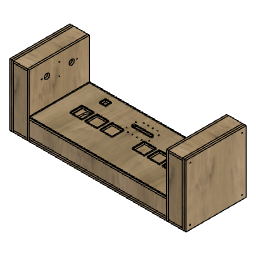
ongekicon-diy (Autodesk Fusion 360 design; units mm, degrees)
Autodesk Fusion 360 part; units mm, degrees
(part 1 of 3)
sketch "스케치1" plane through (0, 0, 0) normal (0, 0, 1) x (1, 0, 0)
  line L0 (289, -642.7336) -> (375, -642.7336)
  line L1 (375, -656.7336) -> (289, -656.7336)
  arc A0 (289, -642.7336) -> (289, -656.7336) centre (289, -649.7336) ccw
  arc A1 (375, -656.7336) -> (375, -642.7336) centre (375, -649.7336) ccw
  line L2 (289, -642.7336) -> (289, -656.7336) construction
  line L3 (375, -642.7336) -> (375, -656.7336) construction
  line L4 (375, -642.7336) -> (386.9217, -626.4866) construction
  line L5 (386.9217, -626.4866) -> (386.9217, -642.6701) construction
  line L6 (386.9217, -642.6701) -> (386.9217, -656.6701) construction
  line L7 (386.9217, -656.6701) -> (386.9217, -672.8535) construction
  line L8 (375, -656.7336) -> (386.9217, -672.8535) construction
  line L9 (386.9217, -642.6701) -> (386.9217, -656.6701) construction
  line L10 (375, -642.7336) -> (375, -656.7336) construction
  line L11 (375, -642.7336) -> (386.9217, -626.4866) construction
  line L12 (375, -656.7336) -> (386.9217, -672.8535) construction
  line L13 (386.9217, -656.6701) -> (386.9217, -672.8535) construction
  line L14 (386.9217, -626.4866) -> (386.9217, -642.6701) construction
  arc A2 (375, -656.7336) -> (375, -642.7336) centre (375, -649.7336) ccw
  line L15 (375, -642.7336) -> (386.9217, -642.7336) construction
  line L16 (289, -642.7336) -> (277.0783, -642.7336) construction
  line L17 (277.0783, -642.7336) -> (277.0783, -626.5501) construction
  line L18 (277.0783, -626.5501) -> (289, -642.7336) construction
  line L19 (289, -656.7336) -> (277.0783, -656.7336) construction
  line L20 (277.0783, -656.7336) -> (277.0783, -672.9171) construction
  line L21 (289, -656.7336) -> (277.0783, -672.9171) construction
  circle A3 centre (277.0783, -626.5501) radius 2.65
  circle A4 centre (277.0783, -672.9171) radius 2.65
  circle A5 centre (386.9217, -626.4866) radius 2.65
  circle A6 centre (386.9217, -672.8535) radius 2.65
  line L22 (299.0783, -611.6097) -> (277.0783, -626.5501) construction
  circle A7 centre (299.0783, -611.6097) radius 2.65
  line L23 (299.0783, -611.6097) -> (321.0783, -611.6097) construction
  line L24 (321.0783, -611.6097) -> (343.0783, -611.6097) construction
  line L25 (343.0783, -611.6097) -> (365.0783, -611.6097) construction
  line L26 (364.9217, -687.7939) -> (386.9217, -672.8535) construction
  line L27 (364.9217, -687.7939) -> (342.9217, -687.7939) construction
  line L28 (342.9217, -687.7939) -> (320.9217, -687.7939) construction
  line L29 (320.9217, -687.7939) -> (298.9217, -687.7939) construction
  circle A8 centre (321.0783, -611.6097) radius 2.65
  circle A9 centre (343.0783, -611.6097) radius 2.65
  circle A10 centre (365.0783, -611.6097) radius 2.65
  circle A11 centre (364.9217, -687.7939) radius 2.65
  circle A12 centre (342.9217, -687.7939) radius 2.65
  circle A13 centre (320.9217, -687.7939) radius 2.65
  circle A14 centre (298.9217, -687.7939) radius 2.65
  line L30 (0, -575) -> (664, -575)
  line L31 (664, -575) -> (664, -866)
  line L32 (664, -866) -> (0, -866)
  line L33 (0, -866) -> (0, -575)
  line L34 (0, -575) -> (332, -575) construction
  line L35 (332, -575) -> (332, -649.7336) construction
  line L36 (0, -649.7336) -> (0, -575) construction
  line L37 (332, -649.7336) -> (289, -649.7336) construction
  line L38 (150.8081, -749.0793) -> (137.915, -749.0793) construction
  line L39 (223.7013, -749.0793) -> (210.8081, -749.0793) construction
  line L40 (842.8371, -502.2992) -> (842.8371, -516.2992) construction
  line L41 (820.8371, -547.4231) -> (842.8371, -532.4827) construction
  line L42 (830.9154, -502.3627) -> (830.9154, -516.3627) construction
  line L43 (830.9154, -516.3627) -> (842.8371, -532.4827) construction
  line L44 (842.8371, -516.2992) -> (842.8371, -532.4827) construction
  circle A15 centre (798.8371, -547.4231) radius 2.65
  circle A16 centre (798.9937, -471.2388) radius 2.65
  line L45 (798.9937, -471.2388) -> (820.9937, -471.2388) construction
  circle A17 centre (820.8371, -547.4231) radius 2.65
  circle A18 centre (842.8371, -532.4827) radius 2.65
  line L46 (820.8371, -547.4231) -> (798.8371, -547.4231) construction
  circle A19 centre (842.8371, -486.1157) radius 2.65
  arc A20 (830.9154, -516.3627) -> (830.9154, -502.3627) centre (830.9154, -509.3627) ccw
  circle A21 centre (820.9937, -471.2388) radius 2.65
  line L47 (830.9154, -502.3627) -> (842.8371, -502.3627) construction
  line L48 (830.9154, -502.3627) -> (830.9154, -516.3627) construction
  line L49 (830.9154, -516.3627) -> (842.8371, -532.4827) construction
  arc A22 (830.9154, -516.3627) -> (830.9154, -502.3627) centre (830.9154, -509.3627) ccw
  line L50 (798.8371, -547.4231) -> (776.8371, -547.4231) construction
  line L51 (744.9154, -502.3627) -> (830.9154, -502.3627)
  line L52 (776.9937, -471.2388) -> (798.9937, -471.2388) construction
  line L53 (830.9154, -516.3627) -> (744.9154, -516.3627)
  circle A23 centre (754.8371, -547.4231) radius 2.65
  line L54 (732.9937, -502.3627) -> (732.9937, -486.1792) construction
  circle A24 centre (776.8371, -547.4231) radius 2.65
  line L55 (787.9154, -509.3627) -> (744.9154, -509.3627) construction
  line L56 (744.9154, -502.3627) -> (732.9937, -502.3627) construction
  line L57 (754.9937, -471.2388) -> (776.9937, -471.2388) construction
  circle A25 centre (776.9937, -471.2388) radius 2.65
  circle A26 centre (754.9937, -471.2388) radius 2.65
  line L58 (732.9937, -486.1792) -> (744.9154, -502.3627) construction
  circle A27 centre (732.9937, -532.5462) radius 2.65
  line L59 (776.8371, -547.4231) -> (754.8371, -547.4231) construction
  line L60 (744.9154, -516.3627) -> (732.9937, -516.3627) construction
  line L61 (732.9937, -516.3627) -> (732.9937, -532.5462) construction
  line L62 (754.9937, -471.2388) -> (732.9937, -486.1792) construction
  line L63 (744.9154, -502.3627) -> (744.9154, -516.3627) construction
  line L64 (830.9154, -502.3627) -> (842.8371, -486.1157) construction
  line L65 (842.8371, -486.1157) -> (842.8371, -502.2992) construction
  line L66 (842.8371, -516.2992) -> (842.8371, -532.4827) construction
  line L67 (842.8371, -486.1157) -> (842.8371, -502.2992) construction
  line L68 (842.8371, -502.2992) -> (842.8371, -516.2992) construction
  line L69 (830.9154, -502.3627) -> (842.8371, -486.1157) construction
  line L70 (744.9154, -516.3627) -> (732.9937, -532.5462) construction
  circle A28 centre (732.9937, -486.1792) radius 2.65
  arc A29 (744.9154, -502.3627) -> (744.9154, -516.3627) centre (744.9154, -509.3627) ccw
  circle A30 centre (-55.9858, -345.9527) radius 2.65
  line L71 (-55.9858, -299.5858) -> (-55.9858, -315.7693) construction
  circle A31 centre (-77.8292, -284.7089) radius 2.65
  line L72 (-153.9075, -329.8328) -> (-165.8292, -346.0163) construction
  line L73 (-121.8292, -284.7089) -> (-99.8292, -284.7089) construction
  line L74 (-153.9075, -329.8328) -> (-165.8292, -329.8328) construction
  arc A32 (-153.9075, -315.8328) -> (-153.9075, -329.8328) centre (-153.9075, -322.8328) ccw
  line L75 (-165.8292, -329.8328) -> (-165.8292, -346.0163) construction
  circle A33 centre (-165.8292, -299.6493) radius 2.65
  circle A34 centre (-143.9858, -360.8931) radius 2.65
  line L76 (-143.8292, -284.7089) -> (-121.8292, -284.7089) construction
  line L77 (-153.9075, -315.8328) -> (-153.9075, -329.8328) construction
  line L78 (-153.9075, -315.8328) -> (-165.8292, -315.8328) construction
  circle A35 centre (-121.8292, -284.7089) radius 2.65
  line L79 (-67.9075, -329.8328) -> (-153.9075, -329.8328)
  line L80 (-55.9858, -315.7693) -> (-55.9858, -329.7693) construction
  line L81 (-153.9075, -315.8328) -> (-67.9075, -315.8328)
  circle A36 centre (-77.9858, -360.8931) radius 2.65
  arc A37 (-67.9075, -329.8328) -> (-67.9075, -315.8328) centre (-67.9075, -322.8328) ccw
  arc A38 (-67.9075, -329.8328) -> (-67.9075, -315.8328) centre (-67.9075, -322.8328) ccw
  line L82 (-67.9075, -315.8328) -> (-55.9858, -299.5858) construction
  line L83 (-67.9075, -315.8328) -> (-67.9075, -329.8328) construction
  line L84 (-67.9075, -315.8328) -> (-55.9858, -315.8328) construction
  circle A39 centre (-55.9858, -299.5858) radius 2.65
  line L85 (-99.8292, -284.7089) -> (-77.8292, -284.7089) construction
  line L86 (-67.9075, -329.8328) -> (-55.9858, -345.9527) construction
  circle A40 centre (-99.9858, -360.8931) radius 2.65
  line L87 (-77.9858, -360.8931) -> (-55.9858, -345.9527) construction
  circle A41 centre (-99.8292, -284.7089) radius 2.65
  line L88 (-55.9858, -299.5858) -> (-55.9858, -315.7693) construction
  line L89 (-67.9075, -329.8328) -> (-55.9858, -345.9527) construction
  line L90 (-77.9858, -360.8931) -> (-99.9858, -360.8931) construction
  line L91 (-55.9858, -329.7693) -> (-55.9858, -345.9527) construction
  line L92 (-55.9858, -329.7693) -> (-55.9858, -345.9527) construction
  line L93 (-165.8292, -315.8328) -> (-165.8292, -299.6493) construction
  line L94 (-165.8292, -299.6493) -> (-153.9075, -315.8328) construction
  line L95 (-99.9858, -360.8931) -> (-121.9858, -360.8931) construction
  line L96 (-110.9075, -322.8328) -> (-153.9075, -322.8328) construction
  circle A42 centre (-165.8292, -346.0163) radius 2.65
  line L97 (-121.9858, -360.8931) -> (-143.9858, -360.8931) construction
  line L98 (-67.9075, -315.8328) -> (-55.9858, -299.5858) construction
  line L99 (-67.9075, -315.8328) -> (-67.9075, -329.8328) construction
  circle A43 centre (-143.8292, -284.7089) radius 2.65
  circle A44 centre (-121.9858, -360.8931) radius 2.65
  line L100 (-55.9858, -315.7693) -> (-55.9858, -329.7693) construction
  line L101 (-143.8292, -284.7089) -> (-165.8292, -299.6493) construction
  line L102 (0, -1260) -> (664, -1260)
  line L103 (664, -1260) -> (664, -1333)
  line L104 (664, -1333) -> (0, -1333)
  line L105 (0, -1333) -> (0, -1260)
  line L106 (0, -1495) -> (0, -1422)
  line L107 (664, -1422) -> (664, -1495)
  line L108 (0, -1422) -> (664, -1422)
  line L109 (664, -1495) -> (0, -1495)
  circle A45 centre (-680.319, -279.9365) radius 2.65
  line L110 (-604.942, -341.2219) -> (-664.942, -341.2219)
  circle A46 centre (-658.319, -264.9961) radius 2.65
  line L111 (-592.0489, -341.2219) -> (-604.942, -341.2219) construction
  line L112 (-834.4326, -341.2219) -> (-834.4326, -281.2219)
  line L113 (-907.3257, -341.2219) -> (-967.3257, -341.2219)
  line L114 (-592.0489, -281.2219) -> (-532.0489, -281.2219)
  line L115 (-967.3257, -281.2219) -> (-907.3257, -281.2219)
  line L116 (-761.5395, -281.2219) -> (-821.5395, -281.2219)
  line L117 (-907.3257, -281.2219) -> (-907.3257, -341.2219)
  line L118 (-821.5395, -341.2219) -> (-834.4326, -341.2219) construction
  line L119 (-532.0489, -341.2219) -> (-592.0489, -341.2219)
  line L120 (-821.5395, -341.2219) -> (-761.5395, -341.2219)
  line L121 (-1045.2407, -198.34) -> (-1045.2407, -167.1425) construction
  line L122 (-821.5395, -281.2219) -> (-821.5395, -341.2219)
  line L123 (-894.4326, -281.2219) -> (-894.4326, -341.2219)
  line L124 (-967.3257, -341.2219) -> (-967.3257, -281.2219)
  circle A47 centre (-724.1625, -203.7522) radius 2.65
  circle A48 centre (-746.1625, -203.7522) radius 2.65
  circle A49 centre (-724.319, -279.9365) radius 2.65
  arc A50 (-756.2407, -234.8761) -> (-756.2407, -248.8761) centre (-756.2407, -241.8761) ccw
  line L125 (-761.5395, -341.2219) -> (-761.5395, -281.2219)
  circle A51 centre (-680.1625, -203.7522) radius 2.65
  line L126 (-592.0489, -341.2219) -> (-592.0489, -281.2219)
  circle A52 centre (-768.1625, -265.0596) radius 2.65
  circle A53 centre (-746.319, -279.9365) radius 2.65
  line L127 (-670.2407, -248.8761) -> (-756.2407, -248.8761)
  circle A54 centre (-768.1625, -218.6926) radius 2.65
  line L128 (-756.2407, -234.8761) -> (-670.2407, -234.8761)
  line L129 (-381.2407, -167.1425) -> (-381.2407, -198.34) construction
  line L130 (-903.551, -198.34) -> (-903.551, -231.34)
  line L131 (-903.551, -231.34) -> (-936.551, -231.34)
  line L132 (-894.4326, -341.2219) -> (-834.4326, -341.2219)
  line L133 (-894.4326, -341.2219) -> (-907.3257, -341.2219) construction
  line L134 (-1045.2407, -241.8761) -> (-1045.2407, -167.1425) construction
  line L135 (-936.551, -198.34) -> (-903.551, -198.34)
  line L136 (-1045.2407, -167.1425) -> (-381.2407, -167.1425)
  line L137 (-1045.2407, -167.1425) -> (-713.2407, -167.1425) construction
  line L138 (-936.551, -231.34) -> (-936.551, -198.34)
  line L139 (-381.2407, -458.1425) -> (-1045.2407, -458.1425)
  line L140 (-1045.2407, -458.1425) -> (-1045.2407, -167.1425)
  line L141 (-834.4326, -281.2219) -> (-894.4326, -281.2219)
  line L142 (-522.9305, -198.34) -> (-522.9305, -231.34)
  line L143 (-519.1557, -281.2219) -> (-519.1557, -341.2219)
  line L144 (-519.1557, -341.2219) -> (-532.0489, -341.2219) construction
  line L145 (-459.1557, -281.2219) -> (-519.1557, -281.2219)
  line L146 (-519.1557, -341.2219) -> (-459.1557, -341.2219)
  line L147 (-489.9305, -231.34) -> (-489.9305, -198.34)
  line L148 (-532.0489, -281.2219) -> (-532.0489, -341.2219)
  line L149 (-489.9305, -198.34) -> (-522.9305, -198.34)
  line L150 (-522.9305, -231.34) -> (-489.9305, -231.34)
  line L151 (-459.1557, -341.2219) -> (-459.1557, -281.2219)
  line L152 (-381.2407, -167.1425) -> (-381.2407, -458.1425)
  circle A55 centre (-658.319, -218.6291) radius 2.65
  line L153 (-664.942, -281.2219) -> (-604.942, -281.2219)
  line L154 (-664.942, -341.2219) -> (-664.942, -281.2219)
  arc A56 (-670.2407, -248.8761) -> (-670.2407, -234.8761) centre (-670.2407, -241.8761) ccw
  circle A57 centre (-702.1625, -203.7522) radius 2.65
  line L155 (-604.942, -281.2219) -> (-604.942, -341.2219)
  circle A58 centre (-702.319, -279.9365) radius 2.65
  arc A59 (-670.2407, -248.8761) -> (-670.2407, -234.8761) centre (-670.2407, -241.8761) ccw
  line L156 (664, 150) -> (664, -141)
  line L157 (0, -141) -> (0, 150)
  line L158 (664, -141) -> (0, -141)
  line L159 (604, 120) -> (60, 120)
  line L160 (634, -81) -> (634, 90)
  line L161 (30, 90) -> (30, -81)
  line L162 (634, 120) -> (30, -111) construction
  line L163 (60, -111) -> (604, -111)
  line L164 (0, 150) -> (664, 150)
  line L165 (30, 120) -> (634, -111) construction
  line L166 (0, 120) -> (0, 150) construction
  line L167 (664, -141) -> (644.0002, -121.0002) construction
  line L168 (664, 150) -> (644.0002, 130.0002) construction
  line L169 (0, 150) -> (19.9998, 130.0002) construction
  line L170 (0, -141) -> (19.9998, -121.0002) construction
  line L171 (664, -491) -> (644.0002, -471.0002) construction
  line L172 (664, -200) -> (644.0002, -219.9998) construction
  line L173 (634, -431) -> (634, -260)
  line L174 (664, -200) -> (664, -491)
  line L175 (30, -230) -> (634, -461) construction
  line L176 (0, -200) -> (664, -200)
  line L177 (60, -461) -> (604, -461)
  line L178 (664, -491) -> (0, -491)
  line L179 (634, -230) -> (30, -461) construction
  line L180 (30, -260) -> (30, -431)
  line L181 (0, -491) -> (19.9998, -471.0002) construction
  line L182 (604, -230) -> (60, -230)
  line L183 (0, -491) -> (0, -200)
  line L184 (0, -200) -> (19.9998, -219.9998) construction
  line L185 (0, -230) -> (0, -200) construction
  arc A60 (60, 120) -> (30, 90) centre (60, 90) ccw
  arc A61 (634, 90) -> (604, 120) centre (604, 90) ccw
  arc A62 (604, -111) -> (634, -81) centre (604, -81) ccw
  arc A63 (30, -81) -> (60, -111) centre (60, -81) ccw
  arc A64 (60, -230) -> (30, -260) centre (60, -260) ccw
  arc A65 (634, -260) -> (604, -230) centre (604, -260) ccw
  arc A66 (604, -461) -> (634, -431) centre (604, -431) ccw
  arc A67 (30, -431) -> (60, -461) centre (60, -431) ccw
  circle A68 centre (644.0002, -219.9998) radius 3.25
  circle A69 centre (644.0002, -471.0002) radius 3.25
  circle A70 centre (644.0002, -121.0002) radius 9
  circle A71 centre (644.0002, 130.0002) radius 9
  circle A72 centre (19.9998, 130.0002) radius 9
  circle A73 centre (19.9998, -121.0002) radius 9
  circle A74 centre (19.9998, -219.9998) radius 3.25
  circle A75 centre (19.9998, -471.0002) radius 3.25
  line L186 (664, -575) -> (644, -575) construction
  line L187 (644, -575) -> (644, -595) construction
  line L188 (644, -595) -> (664, -595) construction
  line L189 (664, -595) -> (664, -575) construction
  line L190 (664, -866) -> (644, -866) construction
  line L191 (644, -866) -> (644, -846) construction
  line L192 (644, -846) -> (664, -846) construction
  line L193 (664, -846) -> (664, -866) construction
  line L194 (0, -866) -> (20, -866) construction
  line L195 (20, -866) -> (20, -846) construction
  line L196 (20, -846) -> (0, -846) construction
  line L197 (0, -846) -> (0, -866) construction
  line L198 (0, -575) -> (20, -575) construction
  line L199 (20, -575) -> (20, -595) construction
  line L200 (20, -595) -> (0, -595) construction
  line L201 (0, -595) -> (0, -575) construction
  circle A76 centre (20, -595) radius 2.5 construction
  circle A77 centre (644, -595) radius 2.5 construction
  circle A78 centre (20, -846) radius 2.5 construction
  circle A79 centre (644, -846) radius 2.5 construction
  line L202 (1066.4968, -1645.2647) -> (1357.4968, -1645.2647)
  line L203 (1357.4968, -1645.2647) -> (1357.4968, -1712.2647)
  line L204 (1357.4968, -1712.2647) -> (1066.4968, -1712.2647)
  line L205 (1066.4968, -1712.2647) -> (1066.4968, -1645.2647)
  line L206 (716.4968, -1645.2647) -> (1007.4968, -1645.2647)
  line L207 (1007.4968, -1645.2647) -> (1007.4968, -1712.2647)
  line L208 (1007.4968, -1712.2647) -> (716.4968, -1712.2647)
  line L209 (716.4968, -1712.2647) -> (716.4968, -1645.2647)
  line L210 (1066.4968, -845.2647) -> (1357.4968, -845.2647)
  line L211 (1357.4968, -845.2647) -> (1357.4968, -912.2647)
  line L212 (1357.4968, -912.2647) -> (1066.4968, -912.2647)
  line L213 (1066.4968, -912.2647) -> (1066.4968, -845.2647)
  line L214 (716.4968, -845.2647) -> (1007.4968, -845.2647)
  line L215 (1007.4968, -845.2647) -> (1007.4968, -912.2647)
  line L216 (1007.4968, -912.2647) -> (716.4968, -912.2647)
  line L217 (716.4968, -912.2647) -> (716.4968, -845.2647)
  line L218 (1406.0943, -1345.433) -> (1473.0943, -1345.433)
  line L219 (1473.0943, -1345.433) -> (1473.0943, -1627.433)
  line L220 (1473.0943, -1627.433) -> (1406.0943, -1627.433)
  line L221 (1406.0943, -1627.433) -> (1406.0943, -1345.433)
  line L222 (1573.0943, -1627.433) -> (1506.0943, -1627.433)
  line L223 (1506.0943, -1627.433) -> (1506.0943, -1345.433)
  line L224 (1506.0943, -1345.433) -> (1573.0943, -1345.433)
  line L225 (1573.0943, -1345.433) -> (1573.0943, -1627.433)
  line L226 (1506.0943, -1277.433) -> (1506.0943, -995.433)
  line L227 (1506.0943, -995.433) -> (1573.0943, -995.433)
  line L228 (1573.0943, -995.433) -> (1573.0943, -1277.433)
  line L229 (1573.0943, -1277.433) -> (1506.0943, -1277.433)
  line L230 (1406.0943, -1277.433) -> (1406.0943, -995.433)
  line L231 (1406.0943, -995.433) -> (1473.0943, -995.433)
  line L232 (1473.0943, -1277.433) -> (1406.0943, -1277.433)
  line L233 (1473.0943, -995.433) -> (1473.0943, -1277.433)
  line L234 (1339.5, -433) -> (1368.5, -433)
  line L235 (1219.5, -433) -> (1248.5, -433)
  line L236 (1248.5, -433) -> (1248.5, -479)
  arc A80 (1370, -497) -> (1385, -482) centre (1370, -482) ccw
  circle A81 centre (1209, -456) radius 2.2592
  line L237 (1203, -415) -> (1385, -497) construction
  arc A82 (1218, -412) -> (1200, -430) centre (1218, -430) ccw
  arc A83 (1218, -415) -> (1203, -430) centre (1218, -430) ccw
  arc A84 (1203, -482) -> (1218, -497) centre (1218, -482) ccw
  line L238 (1218, -497) -> (1370, -497)
  line L239 (1218, -500) -> (1370, -500)
  line L240 (1388, -412) -> (1200, -500) construction
  line L241 (1248.5, -479) -> (1219.5, -479)
  arc A85 (1388, -430) -> (1370, -412) centre (1370, -430) ccw
  circle A86 centre (1294, -486) radius 2.2361
  line L242 (1200, -412) -> (1388, -500) construction
  line L243 (1203, -430) -> (1203, -482)
  line L244 (1370, -415) -> (1218, -415)
  circle A87 centre (1294, -426) radius 2.2361
  line L245 (1370, -412) -> (1218, -412)
  line L246 (1385, -415) -> (1203, -497) construction
  line L247 (1388, -482) -> (1388, -430)
  line L248 (1219.5, -479) -> (1219.5, -433)
  arc A88 (1370, -500) -> (1388, -482) centre (1370, -482) ccw
  arc A89 (1200, -482) -> (1218, -500) centre (1218, -482) ccw
  line L249 (1339.5, -479) -> (1339.5, -433)
  line L250 (1200, -430) -> (1200, -482)
  arc A90 (1385, -430) -> (1370, -415) centre (1370, -430) ccw
  line L251 (1385, -482) -> (1385, -430)
  line L252 (1368.5, -433) -> (1368.5, -479)
  circle A91 centre (1379, -456) radius 2.2361
  line L253 (1368.5, -479) -> (1339.5, -479)
  circle A92 centre (1661.9968, -422.7804) radius 2.2361
  arc A93 (1585.9968, -408.7804) -> (1567.9968, -426.7804) centre (1585.9968, -426.7804) ccw
  line L254 (1587.4968, -429.7804) -> (1616.4968, -429.7804)
  circle A94 centre (1601.9968, -452.7804) radius 12.5
  circle A95 centre (1661.9968, -482.7804) radius 2.2361
  line L255 (1587.4968, -429.7804) -> (1616.4968, -475.7804) construction
  line L256 (1570.9968, -426.7804) -> (1570.9968, -478.7804)
  line L257 (1587.4968, -475.7804) -> (1587.4968, -429.7804)
  line L258 (1616.4968, -475.7804) -> (1587.4968, -475.7804)
  line L259 (1616.4968, -429.7804) -> (1616.4968, -475.7804)
  line L260 (1567.9968, -426.7804) -> (1567.9968, -478.7804)
  line L261 (1516.4968, -587.7804) -> (1516.4968, -660.7804)
  circle A96 centre (1721.9968, -452.7804) radius 12.5
  line L262 (1707.4968, -429.7804) -> (1736.4968, -475.7804) construction
  arc A97 (1752.9968, -426.7804) -> (1737.9968, -411.7804) centre (1737.9968, -426.7804) ccw
  circle A98 centre (1746.9968, -452.7804) radius 2.2361
  line L263 (1707.4968, -475.7804) -> (1707.4968, -429.7804)
  arc A99 (1755.9968, -426.7804) -> (1737.9968, -408.7804) centre (1737.9968, -426.7804) ccw
  arc A100 (1737.9968, -493.7804) -> (1752.9968, -478.7804) centre (1737.9968, -478.7804) ccw
  line L264 (1807.4968, -587.7804) -> (1807.4968, -507.7804) construction
  line L265 (1736.4968, -429.7804) -> (1707.4968, -475.7804) construction
  line L266 (1736.4968, -475.7804) -> (1707.4968, -475.7804)
  arc A101 (1737.9968, -496.7804) -> (1755.9968, -478.7804) centre (1737.9968, -478.7804) ccw
  line L267 (1752.9968, -478.7804) -> (1752.9968, -426.7804)
  line L268 (1707.4968, -429.7804) -> (1736.4968, -429.7804)
  line L269 (1736.4968, -429.7804) -> (1736.4968, -475.7804)
  line L270 (1755.9968, -478.7804) -> (1755.9968, -426.7804)
  circle A102 centre (1576.9968, -452.7804) radius 2.2592
  line L271 (1807.4968, -660.7804) -> (1807.4968, -587.7804)
  arc A103 (1585.9968, -411.7804) -> (1570.9968, -426.7804) centre (1585.9968, -426.7804) ccw
  line L272 (1525.4968, -644.7804) -> (1525.4968, -660.7804) construction
  circle A104 centre (1616.4968, -615.7804) radius 4
  line L273 (1525.4968, -660.7804) -> (1516.4968, -660.7804)
  arc A105 (1570.9968, -626.2804) -> (1574.9968, -630.2804) centre (1570.9968, -630.2804) ccw
  circle A106 centre (1616.4968, -644.7804) radius 4
  line L274 (1585.9968, -496.7804) -> (1737.9968, -496.7804)
  line L275 (1585.9968, -493.7804) -> (1737.9968, -493.7804)
  line L276 (1737.9968, -411.7804) -> (1585.9968, -411.7804)
  line L277 (1807.4968, -378.7804) -> (1516.4968, -378.7804)
  arc A107 (1567.9968, -478.7804) -> (1585.9968, -496.7804) centre (1585.9968, -478.7804) ccw
  arc A108 (1570.9968, -478.7804) -> (1585.9968, -493.7804) centre (1585.9968, -478.7804) ccw
  line L278 (1616.4968, -429.7804) -> (1587.4968, -475.7804) construction
  line L279 (1807.4968, -507.7804) -> (1516.4968, -397.7804) construction
  line L280 (1807.4968, -587.7804) -> (1516.4968, -587.7804)
  line L281 (1737.9968, -408.7804) -> (1585.9968, -408.7804)
  line L282 (1807.4968, -397.7804) -> (1516.4968, -507.7804) construction
  circle A109 centre (1707.4968, -615.7804) radius 4
  line L283 (1516.4968, -660.7804) -> (1807.4968, -660.7804)
  arc A110 (1574.9968, -630.2804) -> (1570.9968, -626.2804) centre (1570.9968, -630.2804) ccw
  circle A111 centre (1707.4968, -644.7804) radius 4
  line L284 (1807.4968, -378.7804) -> (1807.4968, -660.7804)
  line L285 (1516.4968, -378.7804) -> (1516.4968, -660.7804)
  line L286 (1798.4968, -660.7804) -> (1807.4968, -660.7804)
  line L287 (1798.4968, -660.7804) -> (1525.4968, -660.7804)
  circle A112 centre (1661.9968, -630.2804) radius 4
  circle A113 centre (1752.9968, -630.2804) radius 4
  line L288 (725.4968, -1278.433) -> (716.4968, -1278.433)
  line L289 (998.4968, -1278.433) -> (725.4968, -1278.433)
  line L290 (998.4968, -1278.433) -> (1007.4968, -1278.433)
  line L291 (1007.4968, -978.433) -> (1007.4968, -1278.433)
  line L292 (1007.4968, -978.433) -> (716.4968, -978.433)
  line L293 (716.4968, -978.433) -> (716.4968, -1278.433)
  arc A114 (1661.5009, -1535.9592) -> (1691.5009, -1565.9592) centre (1691.5009, -1535.9592) ccw
  line L294 (1871.5009, -1325.9592) -> (1691.5009, -1325.9592)
  arc A115 (1691.5009, -1325.9592) -> (1661.5009, -1355.9592) centre (1691.5009, -1355.9592) ccw
  line L295 (1661.5009, -1355.9592) -> (1661.5009, -1535.9592)
  circle A116 centre (1656.0009, -1571.4592) radius 3.25
  circle A117 centre (1656.0009, -1320.4592) radius 3.25
  line L296 (1636.0009, -1295.9592) -> (1636.0009, -1595.9592)
  arc A118 (2251.5009, -1355.9592) -> (2221.5009, -1325.9592) centre (2221.5009, -1355.9592) ccw
  arc A119 (2221.5009, -1565.9592) -> (2251.5009, -1535.9592) centre (2221.5009, -1535.9592) ccw
  circle A120 centre (2257.0009, -1571.4592) radius 10
  circle A121 centre (2257.0009, -1320.4592) radius 10
  circle A122 centre (2006.0009, -1571.4592) radius 10
  line L297 (2221.5009, -1325.9592) -> (2041.5009, -1325.9592)
  circle A123 centre (2006.0009, -1320.4592) radius 10
  line L298 (2041.5009, -1565.9592) -> (2221.5009, -1565.9592)
  line L299 (2277.0009, -1295.9592) -> (2277.0009, -1595.9592)
  arc A124 (2011.5009, -1535.9592) -> (2041.5009, -1565.9592) centre (2041.5009, -1535.9592) ccw
  arc A125 (2041.5009, -1325.9592) -> (2011.5009, -1355.9592) centre (2041.5009, -1355.9592) ccw
  line L300 (2251.5009, -1535.9592) -> (2251.5009, -1355.9592)
  line L301 (2011.5009, -1355.9592) -> (2011.5009, -1535.9592)
  line L302 (1986.0009, -1295.9592) -> (1986.0009, -1595.9592)
  line L303 (1927.0009, -1295.9592) -> (1927.0009, -1595.9592)
  line L304 (1901.5009, -1535.9592) -> (1901.5009, -1355.9592)
  line L305 (1691.5009, -1565.9592) -> (1871.5009, -1565.9592)
  arc A126 (1871.5009, -1565.9592) -> (1901.5009, -1535.9592) centre (1871.5009, -1535.9592) ccw
  arc A127 (1901.5009, -1355.9592) -> (1871.5009, -1325.9592) centre (1871.5009, -1355.9592) ccw
  circle A128 centre (1907.0009, -1320.4592) radius 3.25
  circle A129 centre (1907.0009, -1571.4592) radius 3.25
  line L306 (1927.0009, -1295.9592) -> (1636.0009, -1295.9592)
  line L307 (1927.0009, -1595.9592) -> (1636.0009, -1595.9592)
  line L308 (2277.0009, -1595.9592) -> (1986.0009, -1595.9592)
  line L309 (2277.0009, -1295.9592) -> (1986.0009, -1295.9592)
  line L310 (1927.0009, -1245.9592) -> (1636.0009, -1245.9592)
  line L311 (1927.0009, -945.9592) -> (1927.0009, -1245.9592)
  line L312 (1661.5009, -1005.9592) -> (1661.5009, -1185.9592)
  line L313 (1636.0009, -945.9592) -> (1636.0009, -1245.9592)
  arc A130 (1901.5009, -1005.9592) -> (1871.5009, -975.9592) centre (1871.5009, -1005.9592) ccw
  circle A131 centre (1907.0009, -1221.4592) radius 3.25
  circle A132 centre (1656.0009, -970.4592) radius 3.25
  circle A133 centre (1907.0009, -970.4592) radius 3.25
  line L314 (2277.0009, -945.9592) -> (2277.0009, -1245.9592)
  line L315 (2041.5009, -1215.9592) -> (2221.5009, -1215.9592)
  line L316 (2277.0009, -945.9592) -> (1986.0009, -945.9592)
  line L317 (1691.5009, -1215.9592) -> (1871.5009, -1215.9592)
  line L318 (1901.5009, -1185.9592) -> (1901.5009, -1005.9592)
  arc A134 (1871.5009, -1215.9592) -> (1901.5009, -1185.9592) centre (1871.5009, -1185.9592) ccw
  line L319 (1871.5009, -975.9592) -> (1691.5009, -975.9592)
  line L320 (1986.0009, -945.9592) -> (1986.0009, -1245.9592)
  circle A135 centre (1656.0009, -1221.4592) radius 3.25
  arc A136 (1661.5009, -1185.9592) -> (1691.5009, -1215.9592) centre (1691.5009, -1185.9592) ccw
  arc A137 (1691.5009, -975.9592) -> (1661.5009, -1005.9592) centre (1691.5009, -1005.9592) ccw
  line L321 (1927.0009, -945.9592) -> (1636.0009, -945.9592)
  arc A138 (2011.5009, -1185.9592) -> (2041.5009, -1215.9592) centre (2041.5009, -1185.9592) ccw
  circle A139 centre (2257.0009, -970.4592) radius 10
  circle A140 centre (2006.0009, -1221.4592) radius 10
  line L322 (2011.5009, -1005.9592) -> (2011.5009, -1185.9592)
  arc A141 (2041.5009, -975.9592) -> (2011.5009, -1005.9592) centre (2041.5009, -1005.9592) ccw
  circle A142 centre (2257.0009, -1221.4592) radius 10
  circle A143 centre (2006.0009, -970.4592) radius 10
  line L323 (2277.0009, -1245.9592) -> (1986.0009, -1245.9592)
  line L324 (2251.5009, -1185.9592) -> (2251.5009, -1005.9592)
  arc A144 (2221.5009, -1215.9592) -> (2251.5009, -1185.9592) centre (2221.5009, -1185.9592) ccw
  line L325 (2221.5009, -975.9592) -> (2041.5009, -975.9592)
  arc A145 (2251.5009, -1005.9592) -> (2221.5009, -975.9592) centre (2221.5009, -1005.9592) ccw
  line L326 (716.4968, -1317.433) -> (716.4968, -1617.433)
  circle A146 centre (801.9968, -1386.933) radius 12.5
  line L327 (1007.4968, -1317.433) -> (716.4968, -1317.433)
  line L328 (1007.4968, -1617.433) -> (716.4968, -1617.433)
  circle A147 centre (921.9968, -1386.933) radius 12.5
  line L329 (716.4968, -1521.933) -> (716.4968, -1617.433)
  circle A148 centre (946.9968, -1386.933) radius 2.2361
  circle A149 centre (776.9968, -1386.933) radius 2.2592
  circle A150 centre (861.9968, -1416.933) radius 2.2361
  line L330 (1007.4968, -1317.433) -> (1007.4968, -1617.433)
  line L331 (1007.4968, -1521.933) -> (716.4968, -1521.933) construction
  circle A151 centre (861.9968, -1356.933) radius 2.2361
  line L332 (716.4968, -1278.433) -> (736.4968, -1278.433) construction
  line L333 (736.4968, -1278.433) -> (736.4968, -1258.433) construction
  line L334 (736.4968, -1258.433) -> (716.4968, -1258.433) construction
  line L335 (716.4968, -1258.433) -> (716.4968, -1278.433) construction
  line L336 (1007.4968, -1278.433) -> (987.4968, -1278.433) construction
  line L337 (987.4968, -1278.433) -> (987.4968, -1258.433) construction
  line L338 (987.4968, -1258.433) -> (1007.4968, -1258.433) construction
  line L339 (1007.4968, -1258.433) -> (1007.4968, -1278.433) construction
  line L340 (1007.4968, -978.433) -> (987.4968, -978.433) construction
  line L341 (987.4968, -978.433) -> (987.4968, -998.433) construction
  line L342 (987.4968, -998.433) -> (1007.4968, -998.433) construction
  line L343 (1007.4968, -998.433) -> (1007.4968, -978.433) construction
  line L344 (716.4968, -978.433) -> (736.4968, -978.433) construction
  line L345 (736.4968, -978.433) -> (736.4968, -998.433) construction
  line L346 (736.4968, -998.433) -> (716.4968, -998.433) construction
  line L347 (716.4968, -998.433) -> (716.4968, -978.433) construction
  circle A152 centre (736.4968, -998.433) radius 2.5
  circle A153 centre (736.4968, -1258.433) radius 2.5
  circle A154 centre (987.4968, -1258.433) radius 2.5
  circle A155 centre (987.4968, -998.433) radius 2.5
  circle A156 centre (1086.4968, -998.433) radius 2.5
  line L348 (1086.4968, -1278.433) -> (1086.4968, -1258.433) construction
  line L349 (1066.4968, -978.433) -> (1066.4968, -1278.433)
  line L350 (1066.4968, -998.433) -> (1066.4968, -978.433) construction
  line L351 (1337.4968, -998.433) -> (1357.4968, -998.433) construction
  line L352 (1337.4968, -1258.433) -> (1357.4968, -1258.433) construction
  line L353 (1066.4968, -1258.433) -> (1066.4968, -1278.433) construction
  line L354 (1086.4968, -1258.433) -> (1066.4968, -1258.433) construction
  circle A157 centre (1086.4968, -1258.433) radius 2.5
  line L355 (1066.4968, -1278.433) -> (1086.4968, -1278.433) construction
  line L356 (1348.4968, -1278.433) -> (1357.4968, -1278.433)
  line L357 (1086.4968, -998.433) -> (1066.4968, -998.433) construction
  line L358 (1066.4968, -978.433) -> (1086.4968, -978.433) construction
  line L359 (1357.4968, -1258.433) -> (1357.4968, -1278.433) construction
  line L360 (1357.4968, -998.433) -> (1357.4968, -978.433) construction
  line L361 (1337.4968, -978.433) -> (1337.4968, -998.433) construction
  line L362 (1348.4968, -1278.433) -> (1075.4968, -1278.433)
  line L363 (1086.4968, -978.433) -> (1086.4968, -998.433) construction
  line L364 (1357.4968, -978.433) -> (1337.4968, -978.433) construction
  line L365 (1357.4968, -978.433) -> (1066.4968, -978.433)
  line L366 (1357.4968, -978.433) -> (1357.4968, -1278.433)
  line L367 (1357.4968, -1278.433) -> (1337.4968, -1278.433) construction
  line L368 (1075.4968, -1278.433) -> (1066.4968, -1278.433)
  circle A158 centre (1337.4968, -1258.433) radius 2.5
  circle A159 centre (1337.4968, -998.433) radius 2.5
  line L369 (1337.4968, -1278.433) -> (1337.4968, -1258.433) construction
  line L370 (0, -1260) -> (166, -1260) construction
  line L371 (166, -1260) -> (166, -1297.5) construction
  line L372 (166, -1297.5) -> (0, -1297.5) construction
  line L373 (0, -1297.5) -> (0, -1260) construction
  line L374 (664, -1260) -> (498, -1260) construction
  line L375 (498, -1260) -> (498, -1297.5) construction
  line L376 (498, -1297.5) -> (664, -1297.5) construction
  line L377 (664, -1297.5) -> (664, -1260) construction
  circle A160 centre (456.3298, -1576.2079) radius 4
  circle A161 centre (547.3298, -1605.2079) radius 4
  line L378 (592.8298, -1576.2079) -> (592.8298, -1605.2079) construction
  circle A162 centre (592.8298, -1590.7079) radius 4
  circle A163 centre (547.3298, -1576.2079) radius 4
  line L379 (410.8298, -1576.2079) -> (592.8298, -1576.2079) construction
  line L380 (365.3298, -1605.2079) -> (365.3298, -1627.2079) construction
  line L381 (410.8298, -1605.2079) -> (365.3298, -1605.2079) construction
  line L382 (410.8298, -1627.2079) -> (410.8298, -1605.2079) construction
  line L383 (410.8298, -1605.2079) -> (410.8298, -1576.2079) construction
  circle A164 centre (410.8298, -1590.7079) radius 4
  circle A165 centre (501.8298, -1590.7079) radius 4
  line L384 (365.3298, -1627.2079) -> (410.8298, -1627.2079) construction
  circle A166 centre (456.3298, -1605.2079) radius 4
  line L385 (592.8298, -1605.2079) -> (410.8298, -1605.2079) construction
  line L386 (50.6704, -1959.5478) -> (50.6704, -1981.5478) construction
  line L387 (278.1704, -1959.5478) -> (96.1704, -1959.5478) construction
  line L388 (96.1704, -1981.5478) -> (96.1704, -1959.5478) construction
  line L389 (96.1704, -1930.5478) -> (278.1704, -1930.5478) construction
  line L390 (278.1704, -1930.5478) -> (323.6704, -1930.5478) construction
  circle A167 centre (232.6704, -1959.5478) radius 4
  line L391 (278.1704, -1930.5478) -> (278.1704, -1959.5478) construction
  circle A168 centre (278.1704, -1945.0478) radius 4
  line L392 (323.6704, -1930.5478) -> (323.6704, -1904.0478) construction
  line L393 (278.1704, -1904.0478) -> (278.1704, -1930.5478) construction
  circle A169 centre (232.6704, -1930.5478) radius 4
  line L394 (323.6704, -1904.0478) -> (278.1704, -1904.0478) construction
  line L395 (96.1704, -1959.5478) -> (50.6704, -1959.5478) construction
  line L396 (96.1704, -1959.5478) -> (96.1704, -1930.5478) construction
  circle A170 centre (141.6704, -1959.5478) radius 4
  circle A171 centre (96.1704, -1945.0478) radius 4
  line L397 (50.6704, -1981.5478) -> (96.1704, -1981.5478) construction
  circle A172 centre (141.6704, -1930.5478) radius 4
  circle A173 centre (187.1704, -1945.0478) radius 4
  line L398 (592.8298, -1576.2079) -> (638.3298, -1576.2079) construction
  line L399 (638.3298, -1576.2079) -> (638.3298, -1554.2079) construction
  line L400 (638.3298, -1554.2079) -> (592.8298, -1554.2079) construction
  line L401 (592.8298, -1554.2079) -> (592.8298, -1576.2079) construction
  line L402 (521.8298, -1571.2079) -> (481.2298, -1571.2079)
  line L403 (479.3298, -1573.1079) -> (479.3298, -1578.7079)
  line L404 (481.8298, -1581.2079) -> (521.8298, -1581.2079)
  line L405 (524.3298, -1578.7079) -> (524.3298, -1573.7079)
  arc A174 (524.3298, -1573.7079) -> (521.8298, -1571.2079) centre (521.8298, -1573.7079) ccw
  arc A175 (521.8298, -1581.2079) -> (524.3298, -1578.7079) centre (521.8298, -1578.7079) ccw
  arc A176 (479.3298, -1578.7079) -> (481.8298, -1581.2079) centre (481.8298, -1578.7079) ccw
  arc A177 (481.2298, -1571.2079) -> (479.3298, -1573.1079) centre (481.2298, -1573.1079) ccw
  line L406 (365.3298, -1554.2079) -> (638.3298, -1554.2079)
  line L407 (638.3298, -1554.2079) -> (638.3298, -1627.2079)
  line L408 (638.3298, -1627.2079) -> (365.3298, -1627.2079)
  line L409 (365.3298, -1627.2079) -> (365.3298, -1554.2079)
  arc A178 (884.4968, -1545.933) -> (881.9968, -1543.433) centre (881.9968, -1545.933) ccw
  line L410 (884.4968, -1550.933) -> (884.4968, -1545.933)
  line L411 (770.9968, -1577.433) -> (770.9968, -1548.433) construction
  line L412 (881.9968, -1543.433) -> (841.3968, -1543.433)
  arc A179 (881.9968, -1553.433) -> (884.4968, -1550.933) centre (881.9968, -1550.933) ccw
  arc A180 (839.4968, -1550.933) -> (841.9968, -1553.433) centre (841.9968, -1550.933) ccw
  circle A181 centre (816.4968, -1577.433) radius 4
  circle A182 centre (861.9968, -1562.933) radius 4
  line L413 (841.9968, -1553.433) -> (881.9968, -1553.433)
  arc A183 (841.3968, -1543.433) -> (839.4968, -1545.333) centre (841.3968, -1545.333) ccw
  circle A184 centre (816.4968, -1548.433) radius 4
  line L414 (952.9968, -1577.433) -> (770.9968, -1577.433) construction
  line L415 (839.4968, -1545.333) -> (839.4968, -1550.933)
  line L416 (770.9968, -1548.433) -> (952.9968, -1548.433) construction
  circle A185 centre (770.9968, -1562.933) radius 4
  circle A186 centre (952.9968, -1562.933) radius 4
  circle A187 centre (907.4968, -1577.433) radius 4
  circle A188 centre (907.4968, -1548.433) radius 4
  line L417 (952.9968, -1548.433) -> (952.9968, -1577.433) construction
  line L418 (952.9968, -1548.433) -> (1007.4968, -1548.433) construction
  line L419 (1007.4968, -1548.433) -> (1007.4968, -1521.933) construction
  line L420 (1007.4968, -1521.933) -> (952.9968, -1521.933) construction
  line L421 (952.9968, -1521.933) -> (952.9968, -1548.433) construction
  line L422 (770.9968, -1577.433) -> (716.4968, -1577.433) construction
  line L423 (716.4968, -1577.433) -> (716.4968, -1594.933) construction
  line L424 (716.4968, -1594.933) -> (770.9968, -1594.933) construction
  line L425 (770.9968, -1594.933) -> (770.9968, -1577.433) construction
  circle A189 centre (1302.9968, -1562.933) radius 4
  circle A190 centre (1257.4968, -1548.433) radius 4
  line L426 (1357.4968, -1521.933) -> (1302.9968, -1521.933) construction
  arc A191 (1231.9968, -1553.433) -> (1234.4968, -1550.933) centre (1231.9968, -1550.933) ccw
  arc A192 (1234.4968, -1545.933) -> (1231.9968, -1543.433) centre (1231.9968, -1545.933) ccw
  line L427 (1120.9968, -1577.433) -> (1120.9968, -1548.433) construction
  line L428 (1231.9968, -1543.433) -> (1191.3968, -1543.433)
  line L429 (1120.9968, -1603.933) -> (1120.9968, -1577.433) construction
  circle A193 centre (1211.9968, -1562.933) radius 4
  line L430 (1302.9968, -1521.933) -> (1302.9968, -1548.433) construction
  line L431 (1302.9968, -1548.433) -> (1302.9968, -1577.433) construction
  circle A194 centre (1257.4968, -1577.433) radius 4
  line L432 (1357.4968, -1317.433) -> (1357.4968, -1617.433)
  line L433 (1302.9968, -1548.433) -> (1357.4968, -1548.433) construction
  line L434 (1357.4968, -1548.433) -> (1357.4968, -1521.933) construction
  arc A195 (1189.4968, -1550.933) -> (1191.9968, -1553.433) centre (1191.9968, -1550.933) ccw
  circle A196 centre (1120.9968, -1562.933) radius 4
  line L435 (1234.4968, -1550.933) -> (1234.4968, -1545.933)
  circle A197 centre (1211.9968, -1356.933) radius 2.2361
  circle A198 centre (1166.4968, -1548.433) radius 4
  arc A199 (1191.3968, -1543.433) -> (1189.4968, -1545.333) centre (1191.3968, -1545.333) ccw
  line L436 (1189.4968, -1545.333) -> (1189.4968, -1550.933)
  circle A200 centre (1166.4968, -1577.433) radius 4
  circle A201 centre (1211.9968, -1416.933) radius 2.2361
  circle A202 centre (1126.9968, -1386.933) radius 2.2592
  line L437 (1191.9968, -1553.433) -> (1231.9968, -1553.433)
  circle A203 centre (1151.9968, -1386.933) radius 12.5
  line L438 (1357.4968, -1617.433) -> (1066.4968, -1617.433)
  line L439 (1120.9968, -1577.433) -> (1066.4968, -1577.433) construction
  line L440 (1066.4968, -1603.933) -> (1120.9968, -1603.933) construction
  line L441 (1066.4968, -1521.933) -> (1066.4968, -1617.433)
  line L442 (1066.4968, -1577.433) -> (1066.4968, -1603.933) construction
  line L443 (1066.4968, -1317.433) -> (1066.4968, -1617.433)
  line L444 (1302.9968, -1577.433) -> (1120.9968, -1577.433) construction
  line L445 (1357.4968, -1317.433) -> (1066.4968, -1317.433)
  line L446 (1120.9968, -1548.433) -> (1302.9968, -1548.433) construction
  line L447 (1357.4968, -1521.933) -> (1066.4968, -1521.933) construction
  circle A204 centre (1296.9968, -1386.933) radius 2.2361
  circle A205 centre (1271.9968, -1386.933) radius 12.5
  line L448 (278.3298, -1554.2079) -> (232.8298, -1554.2079) construction
  line L449 (121.8298, -1581.2079) -> (161.8298, -1581.2079)
  line L450 (161.8298, -1571.2079) -> (121.2298, -1571.2079)
  line L451 (50.8298, -1576.2079) -> (232.8298, -1576.2079) construction
  line L452 (119.3298, -1573.1079) -> (119.3298, -1578.7079)
  line L453 (278.3298, -1554.2079) -> (278.3298, -1627.2079)
  line L454 (232.8298, -1576.2079) -> (232.8298, -1605.2079) construction
  line L455 (278.3298, -1576.2079) -> (278.3298, -1554.2079) construction
  arc A206 (161.8298, -1581.2079) -> (164.3298, -1578.7079) centre (161.8298, -1578.7079) ccw
  arc A207 (119.3298, -1578.7079) -> (121.8298, -1581.2079) centre (121.8298, -1578.7079) ccw
  line L456 (232.8298, -1554.2079) -> (232.8298, -1576.2079) construction
  line L457 (232.8298, -1576.2079) -> (278.3298, -1576.2079) construction
  circle A208 centre (187.3298, -1576.2079) radius 4
  arc A209 (121.2298, -1571.2079) -> (119.3298, -1573.1079) centre (121.2298, -1573.1079) ccw
  line L458 (164.3298, -1578.7079) -> (164.3298, -1573.7079)
  circle A210 centre (187.3298, -1605.2079) radius 4
  circle A211 centre (141.8298, -1590.7079) radius 4
  arc A212 (164.3298, -1573.7079) -> (161.8298, -1571.2079) centre (161.8298, -1573.7079) ccw
  line L459 (278.3298, -1627.2079) -> (5.3298, -1627.2079)
  circle A213 centre (96.3298, -1576.2079) radius 4
  line L460 (232.8298, -1605.2079) -> (50.8298, -1605.2079) construction
  circle A214 centre (232.8298, -1590.7079) radius 4
  line L461 (50.8298, -1605.2079) -> (5.3298, -1605.2079) construction
  line L462 (5.3298, -1627.2079) -> (5.3298, -1554.2079)
  circle A215 centre (50.8298, -1590.7079) radius 4
  line L463 (50.8298, -1627.2079) -> (50.8298, -1605.2079) construction
  line L464 (5.3298, -1627.2079) -> (50.8298, -1627.2079) construction
  line L465 (50.8298, -1605.2079) -> (50.8298, -1576.2079) construction
  circle A216 centre (96.3298, -1605.2079) radius 4
  line L466 (5.3298, -1554.2079) -> (278.3298, -1554.2079)
  line L467 (5.3298, -1605.2079) -> (5.3298, -1627.2079) construction
  line L468 (138.1898, -635.6975) -> (109.1898, -635.6975)
  line L469 (109.1898, -635.6975) -> (109.1898, -606.6975)
  line L470 (109.1898, -606.6975) -> (138.1898, -606.6975)
  line L471 (138.1898, -606.6975) -> (138.1898, -635.6975)
  line L472 (138.1898, -635.6975) -> (109.1898, -606.6975) construction
  line L473 (109.1898, -635.6975) -> (138.1898, -606.6975) construction
  line L474 (525.8102, -635.6975) -> (554.8102, -635.6975)
  line L475 (554.8102, -635.6975) -> (554.8102, -606.6975)
  line L476 (554.8102, -606.6975) -> (525.8102, -606.6975)
  line L477 (525.8102, -606.6975) -> (525.8102, -635.6975)
  line L478 (525.8102, -635.6975) -> (554.8102, -606.6975) construction
  line L479 (554.8102, -635.6975) -> (525.8102, -606.6975) construction
  line L480 (664, -1216) -> (644, -1216) construction
  line L481 (644, -945) -> (664, -945) construction
  circle A217 centre (644, -1196) radius 2.5 construction
  line L482 (644, -1216) -> (644, -1196) construction
  line L483 (554.8102, -985.6975) -> (525.8102, -956.6975) construction
  line L484 (554.8102, -985.6975) -> (554.8102, -956.6975)
  line L485 (664, -925) -> (644, -925) construction
  line L486 (109.1898, -985.6975) -> (109.1898, -956.6975)
  line L487 (0, -925) -> (20, -925) construction
  line L488 (20, -925) -> (20, -945) construction
  line L489 (138.1898, -956.6975) -> (138.1898, -985.6975)
  line L490 (0, -999.7336) -> (0, -925) construction
  line L491 (525.8102, -956.6975) -> (525.8102, -985.6975)
  line L492 (525.8102, -985.6975) -> (554.8102, -956.6975) construction
  line L493 (525.8102, -985.6975) -> (554.8102, -985.6975)
  circle A218 centre (644, -945) radius 2.5 construction
  line L494 (664, -945) -> (664, -925) construction
  line L495 (664, -925) -> (664, -1216)
  line L496 (644, -925) -> (644, -945) construction
  circle A219 centre (20, -1196) radius 2.5 construction
  line L497 (0, -1216) -> (0, -925)
  line L498 (0, -945) -> (0, -925) construction
  line L499 (109.1898, -956.6975) -> (138.1898, -956.6975)
  line L500 (0, -925) -> (332, -925) construction
  line L501 (0, -1216) -> (20, -1216) construction
  line L502 (20, -1196) -> (0, -1196) construction
  line L503 (0, -1196) -> (0, -1216) construction
  line L504 (20, -1216) -> (20, -1196) construction
  arc A220 (289, -992.7336) -> (289, -1006.7336) centre (289, -999.7336) ccw
  arc A221 (375, -1006.7336) -> (375, -992.7336) centre (375, -999.7336) ccw
  arc A222 (375, -1006.7336) -> (375, -992.7336) centre (375, -999.7336) ccw
  line L505 (138.1898, -985.6975) -> (109.1898, -985.6975)
  circle A223 centre (20, -945) radius 2.5 construction
  line L506 (20, -945) -> (0, -945) construction
  line L507 (109.1898, -985.6975) -> (138.1898, -956.6975) construction
  line L508 (138.1898, -985.6975) -> (109.1898, -956.6975) construction
  line L509 (375, -1006.7336) -> (289, -1006.7336)
  line L510 (664, -1216) -> (0, -1216)
  line L511 (0, -925) -> (664, -925)
  line L512 (289, -992.7336) -> (375, -992.7336)
  line L513 (644, -1196) -> (664, -1196) construction
  line L514 (664, -1196) -> (664, -1216) construction
  line L515 (554.8102, -956.6975) -> (525.8102, -956.6975)
  line L516 (644, 525) -> (644, 505) construction
  circle A224 centre (644, 254) radius 2.5
  line L517 (664, 525) -> (644, 525) construction
  line L518 (644, 505) -> (664, 505) construction
  line L519 (664, 254) -> (664, 234) construction
  line L520 (664, 505) -> (664, 525) construction
  circle A225 centre (644, 505) radius 2.5
  line L521 (644, 234) -> (644, 254) construction
  line L522 (664, 234) -> (644, 234) construction
  line L523 (644, 254) -> (664, 254) construction
  line L524 (664, 525) -> (664, 234)
  line L525 (0, 525) -> (332, 525) construction
  line L526 (0, 525) -> (664, 525)
  line L527 (664, 234) -> (0, 234)
  line L528 (0, 234) -> (0, 525)
  line L529 (20, 234) -> (20, 254) construction
  line L530 (20, 254) -> (0, 254) construction
  line L531 (0, 254) -> (0, 234) construction
  line L532 (0, 234) -> (20, 234) construction
  circle A226 centre (20, 254) radius 2.5
  circle A227 centre (20, 505) radius 2.5
  line L533 (0, 525) -> (20, 525) construction
  line L534 (20, 505) -> (0, 505) construction
  line L535 (20, 525) -> (20, 505) construction
  line L536 (0, 505) -> (0, 525) construction
  line L537 (180.5, -1312) -> (151.5, -1312)
  line L538 (151.5, -1312) -> (151.5, -1283)
  line L539 (151.5, -1283) -> (180.5, -1283)
  line L540 (180.5, -1283) -> (180.5, -1312)
  line L541 (180.5, -1312) -> (151.5, -1283) construction
  line L542 (151.5, -1312) -> (180.5, -1283) construction
  line L543 (318.75, -1303.75) -> (306.25, -1303.75)
  line L544 (306.25, -1303.75) -> (306.25, -1291.25)
  line L545 (306.25, -1291.25) -> (318.75, -1291.25)
  line L546 (318.75, -1291.25) -> (318.75, -1303.75)
  line L547 (318.75, -1303.75) -> (306.25, -1291.25) construction
  line L548 (306.25, -1303.75) -> (318.75, -1291.25) construction
  line L549 (332, -1333) -> (332, -1260) construction
  line L550 (483.5, -1312) -> (512.5, -1312)
  line L551 (512.5, -1312) -> (512.5, -1283)
  line L552 (483.5, -1283) -> (483.5, -1312)
  line L553 (512.5, -1283) -> (483.5, -1283)
  line L554 (357.75, -1303.75) -> (357.75, -1291.25)
  line L555 (357.75, -1291.25) -> (345.25, -1291.25)
  line L556 (345.25, -1303.75) -> (357.75, -1303.75)
  line L557 (345.25, -1291.25) -> (345.25, -1303.75)
  line L558 (136.915, -748.0793) -> (78.915, -748.0793)
  line L559 (78.915, -748.0793) -> (78.915, -690.0793)
  line L560 (78.915, -690.0793) -> (136.915, -690.0793)
  line L561 (136.915, -690.0793) -> (136.915, -748.0793)
  line L562 (136.915, -748.0793) -> (78.915, -690.0793) construction
  line L563 (78.915, -748.0793) -> (136.915, -690.0793) construction
  line L564 (209.8081, -748.0793) -> (151.8081, -748.0793)
  line L565 (151.8081, -748.0793) -> (151.8081, -690.0793)
  line L566 (151.8081, -690.0793) -> (209.8081, -690.0793)
  line L567 (209.8081, -690.0793) -> (209.8081, -748.0793)
  line L568 (209.8081, -748.0793) -> (151.8081, -690.0793) construction
  line L569 (151.8081, -748.0793) -> (209.8081, -690.0793) construction
  line L570 (282.7013, -748.0793) -> (224.7013, -748.0793)
  line L571 (224.7013, -748.0793) -> (224.7013, -690.0793)
  line L572 (224.7013, -690.0793) -> (282.7013, -690.0793)
  line L573 (282.7013, -690.0793) -> (282.7013, -748.0793)
  line L574 (282.7013, -748.0793) -> (224.7013, -690.0793) construction
  line L575 (224.7013, -748.0793) -> (282.7013, -690.0793) construction